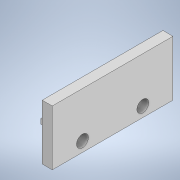
# Autodesk Inventor part: USB_MOUNT
Saved by Autodesk Inventor 2021 (Build 250183000, 183)
## iProperties
Created: 2021-04-21
Part Number: USB_MOUNT
Material: Generic
Document SubType Name: Modeling
Designer: Patrick
Density: 1 g/cm^3
Appearance: Default
Author: Patrick
Autodesk Inventor part; units mm, degrees
ref_plane "YZ Plane" through (0, 0, 0) normal (1, 0, 0) x (0, 1, 0)
ref_plane "XZ Plane" through (0, 0, 0) normal (0, 1, 0) x (-1, 0, 0)
ref_plane "XY Plane" through (0, 0, 0) normal (0, 0, 1) x (1, 0, 0)
sketch "Sketch1" plane through (0, 0, 0) normal (0, 1, 0) x (-1, 0, 0)
  circle A0 centre (0, -5.8) radius 1.45
  circle A1 centre (0, 0) radius 1.45
  line L0 (-1.45, -5.923) -> (-1.45, 0.123)
  line L1 (1.45, 0.123) -> (1.45, -5.923)
  circle A2 centre (0, -5.8) radius 1.45
  circle A3 centre (0, 0) radius 1.45
  line L2 (-1.45, -5.923) -> (-1.45, 0.123)
  line L3 (1.45, -5.923) -> (1.45, 0.123)
  line L4 (-1.45, -5.923) -> (1.45, -0.0104)
  line L5 (1.45, -5.923) -> (-1.45, -0.0056)
  line L6 (5.87, 3.81) -> (-3.02, 3.81)
  line L7 (-3.02, 3.81) -> (-3.02, -9.3582)
  line L8 (5.87, -9.3582) -> (5.87, 3.81)
  line L9 (0, -5.8) -> (0, -9.61)
  line L10 (5.87, -9.3582) -> (5.87, -9.61)
  line L11 (5.87, -9.61) -> (0, -9.61)
  line L12 (-3.02, -9.61) -> (-3.02, -9.3582)
  line L13 (0, -9.61) -> (-3.02, -9.61)
  point P0 (3.8566, 2.9938)
  point P1 (-1.4456, -5.9139)
  point P2 (-1.45, -5.8099)
  point P3 (-1.45, -5.7901)
  point P4 (-1.45, -0.0056)
  point P5 (1.45, -0.0104)
  point P6 (1.45, -5.7873)
  point P7 (1.45, -5.8126)
  point P8 (1.4456, -5.9139)
  dimension "d4" = 0
  dimension "d5" = 2.9
  dimension "d6" = 2.9001
  dimension "d8" = 1.57
  dimension "d9" = 8.89
  dimension "d11" = 3.81
  dimension "d13" = 3.81
  constraints: 26 end point, 4 centre point, 4 perpendicular, 3 coincident, 3 point on line, 2 concentric, 2 parallel, 2 point on circle, 2 vertical, 1 collinear, 1 horizontal, 3 other
  measures "d4" horizontal distance of A0.centre A1.centre
  measures "d5" diameter of A1
  measures "d6" diameter of A0
  measures "d8" distance from line of L5.end L7
  measures "d9" distance between parallel lines of L8 L7
  measures "d11" distance from line of L6 point (0, 0)
  measures "d13" distance of L9.start L9.end
extrude "Extrusion1" add sketch "Sketch1" along normal blind 1.27
sketch "Sketch2" plane through (3.02, 0, 3.81) normal (1, 0, 0) x (0, 0, -1)
  line L0 (9.6001, 1.27) -> (3.8156, 1.27) projected
  line L1 (3.8204, 1.27) -> (9.5973, 1.27) projected
  line L2 (2.36, 1.27) -> (3.8204, 1.27) projected
  line L3 (9.7239, 1.27) -> (11.06, 1.27) projected
  line L4 (6.71, 0) -> (6.71, 13.97)
  line L5 (6.71, 13.97) -> (21.95, 13.97)
  line L6 (21.95, 13.97) -> (21.95, 0)
  line L7 (21.95, 0) -> (6.71, 0)
  line L8 (6.71, 0) -> (6.71, 13.97)
  line L9 (6.71, 13.97) -> (-8.53, 13.97)
  line L10 (-8.53, 13.97) -> (-8.53, 0)
  line L11 (-8.53, 0) -> (6.71, 0)
  line L12 (6.71, 0) -> (6.71, 13.97)
  line L13 (0, 0) -> (13.42, 0) projected
  line L14 (13.42, 0) -> (13.42, 1.27) projected
  line L15 (0, 1.27) -> (13.42, 1.27) projected
  line L16 (0, 0) -> (0, 1.27) projected
  circle A0 centre (14.33, 2.5137) radius 1.5
  circle A1 centre (-0.91, 2.5137) radius 1.5
  point P0 (3.81, 0)
  point P1 (9.7239, 1.27)
  dimension "d19" = 15.24
  dimension "d20" = 15.24
  dimension "d21" = 7.62
  dimension "d22" = 7.62
  dimension "d23" = 3
  dimension "d24" = 3
  constraints: 18 end point, 4 parallel, 2 centre point, 2 horizontal, 2 perpendicular, 1 point on line
  measures "d19" distance of L6.end L7.end
  measures "d20" distance of L11.end L10.end
  measures "d21" distance from line of L4 A0.centre
  measures "d22" distance from line of A1.centre L4
  measures "d23" diameter of A0
  measures "d24" diameter of A1
extrude "Extrusion2" add sketch "Sketch2" along normal blind 2.54
body "Solid1"
